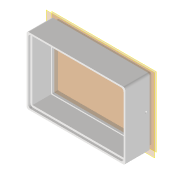
# Autodesk Inventor part: NematostellaImager_spacer_v0
Saved by Autodesk Inventor 2022.5 (Build 265521000, 521)
## iProperties
Created: 2023-11-15
Part Number: NematostellaImager_spacer_v0
Material: Generisch
Document SubType Name: Modeling
Designer: diederichbenedict
Density: 1 g/cm^3
Appearance: Vorgabe
Author: diederichbenedict
Autodesk Inventor part; units mm, degrees
ref_plane "YZ Plane" through (0, 0, 0) normal (1, 0, 0) x (0, 1, 0)
ref_plane "XZ Plane" through (0, 0, 0) normal (0, 1, 0) x (-1, 0, 0)
ref_plane "Arbeitsebene1" through (0, 0, 0) normal (0, 0, 1) x (1, 0, 0)
ref_plane "Arbeitsebene2" through (0, 0, 5) normal (0, 0, 1) x (1, 0, 0)
sketch "Skizze2" plane through (0, 0, 5) normal (0, 0, 1) x (1, 0, 0)
  arc A0 (-24.056, -76.2783) -> (-18.8, -75.35) centre (-21.51, -75.35) ccw projected
  arc A1 (63.445, -45.3) -> (66.445, -42.3) centre (63.445, -42.3) ccw projected
  line L0 (66.445, -42.3) -> (66.445, 42.3) projected
  arc A2 (66.445, 42.3) -> (63.445, 45.3) centre (63.445, 42.3) ccw projected
  line L1 (63.445, 45.3) -> (-63.445, 45.3) projected
  arc A3 (-63.445, 45.3) -> (-66.445, 42.3) centre (-63.445, 42.3) ccw projected
  line L2 (-66.445, 42.3) -> (-66.445, -42.3) projected
  arc A4 (-66.445, -42.3) -> (-63.445, -45.3) centre (-63.445, -42.3) ccw projected
  line L3 (-63.445, -45.3) -> (63.445, -45.3) projected
  arc A5 (63.945, 39.8) -> (60.945, 42.8) centre (60.945, 39.8) ccw projected
  line L4 (63.945, 39.8) -> (63.945, -39.8) projected
  arc A6 (60.945, -42.8) -> (63.945, -39.8) centre (60.945, -39.8) ccw projected
  line L5 (60.945, -42.8) -> (-60.945, -42.8) projected
  arc A7 (-63.945, -39.8) -> (-60.945, -42.8) centre (-60.945, -39.8) ccw projected
  line L6 (-63.945, -39.8) -> (-63.945, 39.8) projected
  arc A8 (-60.945, 42.8) -> (-63.945, 39.8) centre (-60.945, 39.8) ccw projected
  line L7 (-60.945, 42.8) -> (60.945, 42.8) projected
  line L8 (-61.945, 39.8) -> (-61.945, -39.8)
  arc A9 (-61.945, -39.8) -> (-60.945, -40.8) centre (-60.945, -39.8) ccw
  line L9 (-60.945, -40.8) -> (60.945, -40.8)
  arc A10 (60.945, -40.8) -> (61.945, -39.8) centre (60.945, -39.8) ccw
  line L10 (61.945, -39.8) -> (61.945, 39.8)
  arc A11 (61.945, 39.8) -> (60.945, 40.8) centre (60.945, 39.8) ccw
  line L11 (60.945, 40.8) -> (-60.945, 40.8)
  arc A12 (-60.945, 40.8) -> (-61.945, 39.8) centre (-60.945, 39.8) ccw
  point P0 (0, 0)
  dimension "d1" = 2
  constraints: 8 end point, 8 point on circle, 4 centre point, 7 other
  measures "d1" distance between parallel lines of L6 L8
ref_plane "Arbeitsebene3" through (-63.945, -42.8, 0) normal (0, 0, 1) x (1, 0, 0)
extrude "Extrusion1" add sketch "Skizze2" against normal up to surface (5 mm away) draft -2 contours L4 A6 L5 A7 L6 A8 L7 A5
sketch "Skizze3" plane through (0, 0, 5) normal (0, 0, 1) x (1, 0, 0)
  arc A0 (63.445, -45.3) -> (66.445, -42.3) centre (63.445, -42.3) ccw projected
  line L0 (66.445, -42.3) -> (66.445, 42.3) projected
  arc A1 (66.445, 42.3) -> (63.445, 45.3) centre (63.445, 42.3) ccw projected
  line L1 (63.445, 45.3) -> (-63.445, 45.3) projected
  arc A2 (-63.445, 45.3) -> (-66.445, 42.3) centre (-63.445, 42.3) ccw projected
  line L2 (-66.445, 42.3) -> (-66.445, -42.3) projected
  arc A3 (-66.445, -42.3) -> (-63.445, -45.3) centre (-63.445, -42.3) ccw projected
  line L3 (-63.445, -45.3) -> (63.445, -45.3) projected
  arc A4 (63.945, 39.8) -> (60.945, 42.8) centre (60.945, 39.8) ccw projected
  line L4 (63.945, 39.8) -> (63.945, -39.8) projected
  arc A5 (60.945, -42.8) -> (63.945, -39.8) centre (60.945, -39.8) ccw projected
  line L5 (60.945, -42.8) -> (-60.945, -42.8) projected
  arc A6 (-63.945, -39.8) -> (-60.945, -42.8) centre (-60.945, -39.8) ccw projected
  line L6 (-63.945, -39.8) -> (-63.945, 39.8) projected
  arc A7 (-60.945, 42.8) -> (-63.945, 39.8) centre (-60.945, 39.8) ccw projected
  line L7 (-60.945, 42.8) -> (60.945, 42.8) projected
  line L8 (-61.945, -39.8) -> (-61.945, 39.8) projected
  arc A8 (-60.945, 40.8) -> (-61.945, 39.8) centre (-60.945, 39.8) ccw projected
  line L9 (-60.945, 40.8) -> (60.945, 40.8) projected
  arc A9 (61.945, 39.8) -> (60.945, 40.8) centre (60.945, 39.8) ccw projected
  line L10 (61.945, 39.8) -> (61.945, -39.8) projected
  arc A10 (60.945, -40.8) -> (61.945, -39.8) centre (60.945, -39.8) ccw projected
  line L11 (60.945, -40.8) -> (-60.945, -40.8) projected
  arc A11 (-61.945, -39.8) -> (-60.945, -40.8) centre (-60.945, -39.8) ccw projected
  line L12 (63.945, -39.8) -> (63.945, 39.8) projected
  arc A12 (63.945, 39.8) -> (60.945, 42.8) centre (60.945, 39.8) ccw projected
  line L13 (60.945, 42.8) -> (-60.945, 42.8) projected
  arc A13 (-60.945, 42.8) -> (-63.945, 39.8) centre (-60.945, 39.8) ccw projected
  line L14 (-63.945, 39.8) -> (-63.945, -39.8) projected
  arc A14 (-63.945, -39.8) -> (-60.945, -42.8) centre (-60.945, -39.8) ccw projected
  line L15 (-60.945, -42.8) -> (60.945, -42.8) projected
  arc A15 (60.945, -42.8) -> (63.945, -39.8) centre (60.945, -39.8) ccw projected
  point P0 (0, 0)
extrude "Extrusion2" add sketch "Skizze3" along normal blind 3 contours L3 A3 L2 A2 L1 A1 L0 A0 | L4 A5 L5 A6 L6 A7 L7 A4
sketch "Skizze4" plane through (0, 0, 8) normal (0, 0, 1) x (1, 0, 0)
  line L0 (66.445, -42.3) -> (66.445, 42.3) projected
  arc A0 (66.445, 42.3) -> (63.445, 45.3) centre (63.445, 42.3) ccw projected
  line L1 (63.445, 45.3) -> (-63.445, 45.3) projected
  arc A1 (-63.445, 45.3) -> (-66.445, 42.3) centre (-63.445, 42.3) ccw projected
  line L2 (-66.445, 42.3) -> (-66.445, -42.3) projected
  arc A2 (-66.445, -42.3) -> (-63.445, -45.3) centre (-63.445, -42.3) ccw projected
  line L3 (-63.445, -45.3) -> (63.445, -45.3) projected
  arc A3 (63.445, -45.3) -> (66.445, -42.3) centre (63.445, -42.3) ccw projected
  line L4 (60.945, -40.8) -> (-60.945, -40.8) projected
  arc A4 (-61.945, -39.8) -> (-60.945, -40.8) centre (-60.945, -39.8) ccw projected
  line L5 (-61.945, -39.8) -> (-61.945, 39.8) projected
  arc A5 (-60.945, 40.8) -> (-61.945, 39.8) centre (-60.945, 39.8) ccw projected
  line L6 (-60.945, 40.8) -> (60.945, 40.8) projected
  arc A6 (61.945, 39.8) -> (60.945, 40.8) centre (60.945, 39.8) ccw projected
  line L7 (61.945, 39.8) -> (61.945, -39.8) projected
  arc A7 (60.945, -40.8) -> (61.945, -39.8) centre (60.945, -39.8) ccw projected
  line L8 (-63.445, -42.3) -> (-63.445, 42.3)
  line L9 (-63.445, 42.3) -> (63.445, 42.3)
  line L10 (63.445, 42.3) -> (63.445, -42.3)
  line L11 (63.445, -42.3) -> (-63.445, -42.3)
  point P0 (0, 0)
  dimension "d6" = 3
  constraints: 8 end point, 3 other
  measures "d6" distance between parallel lines of L2 L8
extrude "Extrusion3" add sketch "Skizze4" along normal blind 25 contours A3 L3 A2 L2 A1 L1 A0 L0
sketch "Skizze5" plane through (0, 0, 33) normal (0, 0, 1) x (1, 0, 0)
  arc A0 (66.445, 42.3) -> (63.445, 45.3) centre (63.445, 42.3) ccw projected
  line L0 (63.445, 45.3) -> (-63.445, 45.3) projected
  arc A1 (-63.445, 45.3) -> (-66.445, 42.3) centre (-63.445, 42.3) ccw projected
  line L1 (-66.445, 42.3) -> (-66.445, -42.3) projected
  arc A2 (-66.445, -42.3) -> (-63.445, -45.3) centre (-63.445, -42.3) ccw projected
  line L2 (-63.445, -45.3) -> (63.445, -45.3) projected
  arc A3 (63.445, -45.3) -> (66.445, -42.3) centre (63.445, -42.3) ccw projected
  line L3 (66.445, -42.3) -> (66.445, 42.3) projected
  line L4 (-63.445, -42.3) -> (-63.445, 42.3) projected
  line L5 (-63.445, 42.3) -> (63.445, 42.3) projected
  line L6 (63.445, 42.3) -> (63.445, -42.3) projected
  line L7 (63.445, -42.3) -> (-63.445, -42.3) projected
  line L8 (-61.445, -40.3) -> (-61.445, 40.3)
  line L9 (-61.445, 40.3) -> (61.445, 40.3)
  line L10 (61.445, 40.3) -> (61.445, -40.3)
  line L11 (61.445, -40.3) -> (-61.445, -40.3)
  point P0 (0, 0)
  dimension "d9" = 2
  constraints: 8 end point, 3 other
  measures "d9" distance between parallel lines of L7 L11
extrude "Extrusion4" add sketch "Skizze5" along normal blind 2 contours L3 A3 L2 A2 L1 A1 L0 A0 | L4 L5 L6 L7
sketch "Skizze6" plane through (0, 0, 35) normal (0, 0, 1) x (1, 0, 0)
  line L0 (-60.625, -42.48) -> (60.625, -42.48) projected
  arc A0 (-63.625, -39.48) -> (-60.625, -42.48) centre (-60.625, -39.48) ccw projected
  line L1 (-63.625, 39.48) -> (-63.625, -39.48) projected
  arc A1 (-60.625, 42.48) -> (-63.625, 39.48) centre (-60.625, 39.48) ccw projected
  line L2 (60.625, 42.48) -> (-60.625, 42.48) projected
  arc A2 (63.625, 39.48) -> (60.625, 42.48) centre (60.625, 39.48) ccw projected
  line L3 (63.625, -39.48) -> (63.625, 39.48) projected
  arc A3 (60.625, -42.48) -> (63.625, -39.48) centre (60.625, -39.48) ccw projected
  line L4 (53.1911, 40.1013) -> (61.2463, 32.0461) projected
  arc A4 (53.1911, 40.1013) -> (51.0698, 40.98) centre (51.0698, 37.98) ccw projected
  line L5 (51.0698, 40.98) -> (-59.125, 40.98) projected
  arc A5 (-59.125, 40.98) -> (-62.125, 37.98) centre (-59.125, 37.98) ccw projected
  line L6 (-62.125, 37.98) -> (-62.125, -37.98) projected
  arc A6 (-62.125, -37.98) -> (-59.125, -40.98) centre (-59.125, -37.98) ccw projected
  line L7 (-59.125, -40.98) -> (51.0698, -40.98) projected
  arc A7 (51.0698, -40.98) -> (53.1911, -40.1013) centre (51.0698, -37.98) ccw projected
  line L8 (61.2463, -32.0461) -> (53.1911, -40.1013) projected
  arc A8 (61.2463, -32.0461) -> (62.125, -29.9248) centre (59.125, -29.9248) ccw projected
  line L9 (62.125, -29.9248) -> (62.125, 29.9248) projected
  arc A9 (62.125, 29.9248) -> (61.2463, 32.0461) centre (59.125, 29.9248) ccw projected
  arc A10 (-64.125, -39.48) -> (-60.625, -42.98) centre (-60.625, -39.48) ccw
  line L10 (-60.625, -42.98) -> (60.625, -42.98)
  arc A11 (60.625, -42.98) -> (64.125, -39.48) centre (60.625, -39.48) ccw
  line L11 (64.125, -39.48) -> (64.125, 39.48)
  arc A12 (64.125, 39.48) -> (60.625, 42.98) centre (60.625, 39.48) ccw
  line L12 (60.625, 42.98) -> (-60.625, 42.98)
  arc A13 (-60.625, 42.98) -> (-64.125, 39.48) centre (-60.625, 39.48) ccw
  line L13 (-64.125, 39.48) -> (-64.125, -39.48)
  line L14 (63.445, 45.3) -> (-63.445, 45.3) projected
  arc A14 (-63.445, 45.3) -> (-66.445, 42.3) centre (-63.445, 42.3) ccw projected
  line L15 (-66.445, 42.3) -> (-66.445, -42.3) projected
  arc A15 (-66.445, -42.3) -> (-63.445, -45.3) centre (-63.445, -42.3) ccw projected
  line L16 (-63.445, -45.3) -> (63.445, -45.3) projected
  arc A16 (63.445, -45.3) -> (66.445, -42.3) centre (63.445, -42.3) ccw projected
  line L17 (66.445, -42.3) -> (66.445, 42.3) projected
  arc A17 (66.445, 42.3) -> (63.445, 45.3) centre (63.445, 42.3) ccw projected
  line L18 (-61.445, -40.3) -> (-61.445, 40.3) projected
  line L19 (-61.445, 40.3) -> (61.445, 40.3) projected
  line L20 (61.445, 40.3) -> (61.445, -40.3) projected
  line L21 (61.445, -40.3) -> (-61.445, -40.3) projected
  point P0 (0, 0)
  dimension "d12" = 0.5
  constraints: 8 end point, 8 point on circle, 4 centre point, 7 other
  measures "d12" distance between parallel lines of L1 L13
extrude "Extrusion5" add sketch "Skizze6" along normal blind 3 contours A17 L17 A16 L16 A15 L15 A14 L14
sketch "Skizze7" plane through (66.445, -42.3, 5) normal (1, 0, 0) x (0, 0, -1)
  circle A0 centre (-5.052, 45.2732) radius 1.49 projected
  circle A1 centre (-20.052, 60.2732) radius 1.4 projected
  point P0 (5, 42.3)
hole "Bohrung1" at (66.445, 2.9732, 10.052) at (66.445, 17.9732, 25.052) direction (-1, 0, 0) diameter 2.8 end through all
